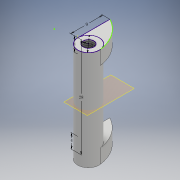
# Autodesk Inventor part: 零件1
Saved by Autodesk Inventor 2018.2 (Build 222227000, 227)
## iProperties
Created: 2017-12-27
Part Number: 零件1
Material: 常规
Document SubType Name: Modeling
Designer: Administrator
Density: 1 g/cm^3
Appearance: 默认
Author: Administrator
Autodesk Inventor part; units mm, degrees
ref_plane "YZ Plane" through (0, 0, 0) normal (1, 0, 0) x (0, 1, 0)
ref_plane "XZ Plane" through (0, 0, 0) normal (0, 1, 0) x (-1, 0, 0)
sketch "草图1" plane through (0, 0, 0) normal (0, 0, 1) x (1, 0, 0)
  circle A0 centre (0, 0) radius 1.5
  circle A1 centre (0, 0) radius 3
  line L0 (-3, 0) -> (-3, 9)
  arc A2 (2.9736, 0.3973) -> (-3, 9) centre (-8.3955, -1.1218) ccw
  dimension "d0" = 3
  dimension "d1" = 6
  dimension "d2" = 9
  constraints: 4 point on circle, 3 centre point, 2 coincident, 2 end point, 2 tangent, 1 vertical
  measures "d0" diameter of A0
  measures "d1" diameter of A1
  measures "d2" distance of L0.start L0.end
sketch "草图2" plane through (0, 0, 0) normal (0, 1, 0) x (-1, 0, 0)
  line L0 (3, 0) -> (3, -28)
  line L1 (3, 0) -> (3, -4)
  line L2 (3, -28) -> (3, -24)
  point P0 (0, 0)
  point P1 (3, -14)
  dimension "d3" = 28
  dimension "d6" = 4
  dimension "d7" = 4
  constraints: 6 end point, 2 point on line, 1 midpoint, 1 vertical
  measures "d3" distance of L0.start L0.end
  measures "d6" distance of L0.start L1.end
  measures "d7" distance of L0.end L2.end
extrude "拉伸1" add sketch "草图1" against normal blind 28 contours A1
extrude "拉伸2" add sketch "草图1" against normal blind 4 contours A1 L0 A2
ref_plane "工作平面1" through (0, 0, -14) normal (0, 0, 1) x (1, 0, 0)
mirror "镜像1" about plane through (0, 0, -14) normal (0, 0, 1) of "拉伸2"
thread "螺纹8" size "M3x0.5" class "6H" standard "ANSI Metric M Profile" full length
